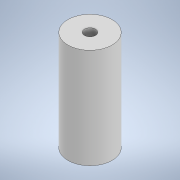
# Autodesk Inventor part: pieza base de bobina
Saved by Autodesk Inventor 2020 (Build 240168000, 168)
## iProperties
Created: 2022-10-18
Part Number: pieza base de bobina
Material: Genérico
Document SubType Name: Modeling
Designer: General
Density: 1 g/cm^3
Appearance: Valor por defecto
Author: General
Autodesk Inventor part; units mm, degrees
ref_plane "YZ Plane" through (0, 0, 0) normal (1, 0, 0) x (0, 1, 0)
ref_plane "XZ Plane" through (0, 0, 0) normal (0, 1, 0) x (-1, 0, 0)
ref_plane "XY Plane" through (0, 0, 0) normal (0, 0, 1) x (1, 0, 0)
sketch "Boceto1" plane through (0, 0, 0) normal (0, 1, 0) x (-1, 0, 0)
  circle A0 centre (0, 0) radius 9.9365
  constraints: 1 centre point, 1 coincident
extrude "Extrusión1" add sketch "Boceto1" along normal blind 30
extrude "Extrusión2" cut sketch "Boceto1" along normal blind 30
extrude "Extrusión3" add sketch "Boceto1" along normal blind 45
sketch "Boceto2" plane through (0, 45, 0) normal (0, 1, 0) x (1, 0, 0)
  point P0 (0, 0)
hole "Agujero1" at (0, 45, 0) direction (0, -1, 0) diameter 5 end through all
